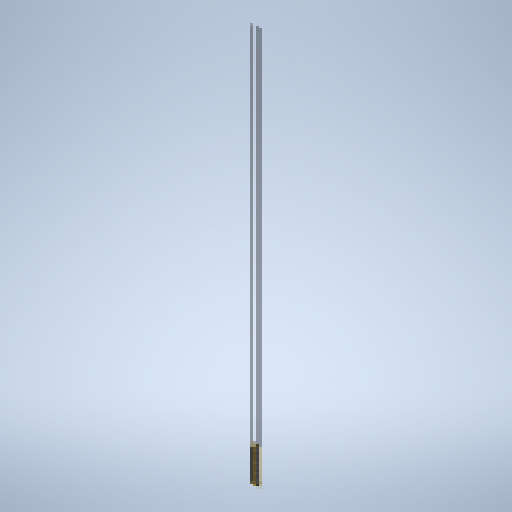
# Autodesk Inventor part: PP0735H(1)
Saved by Autodesk Inventor 2025.2 (Build 292293000, 293)
## iProperties
Category: PARTsolutions
Company: ELDON
Created: 2025-05-02
Part Number: PP0735H(1)
Material: Generic
Catalog Web Link: www.cadenas.de
Description: PP-DIN rails
Vendor: ELDON
Document SubType Name: Modeling
Designer: psAdmin
Manufacturer: ELDON
Mass: 630 g
Surface Area: 1764.71 cm^2
Volume: 84.5125 cm^3
Density: 1 g/cm^3
Appearance: PSOLRGB-175-175-175
PSOL_IDENT_0: {$CADENAS_DATA/23d-libs/eldon/common_pool/accessories/p/pp.prj},167 {VTYP=3D},{NB=PP0735H(1)},{LINA=
PSOL_IDENT_1: PP0735H},{NN=PP},{DATE=04.03.2025 09:38:01},{GEOMDATE=28.02.2025 11:58:07},{VERSION=},{LINEID=1810},
PSOL_IDENT_2: {WBVAR=DETAIL},{WBNUMERIC=DETAIL}  {NB=PP0735H(1)},{LINA=PP0735H},{KT=DUMMY},{ITEM=PP0735H},{DETAIL=
PSOL_IDENT_3: 1},{INFO=Info URL},{DES=Din rail with holes, 2000},{DES1=With holes},{MAT=Galvanized steel},{TYP=Ome
PSOL_IDENT_4: ga},{DIM=7.5 X 35},{HP=Hole pattern 18 x 5.2 mm},{MASS=0.63},{EAN=8713574013193},{TARIFFN=-},{MI=URL
PSOL_IDENT_5: },{MIALG=https://www.eldon.com/catalog-document/PP0515H/mountinginstructions/en/},{INFOPATH=https://
PSOL_IDENT_6: www.nvent.com/en-gb/catalog-document/itemsheet?pid=PP0735H},{V=1},{A=35},{A1=7.5},{A2=4.00},{A3=0.8}
PSOL_IDENT_7: ,{A4=1.8},{A5=0.00},{A6=0.0}
NB: PP0735H(1)
NN: PP
NT: DIN rails
NBSYN: $ITEM.($DETAIL.)
LINA: PP0735H
CATALOG: nVent HOFFMAN IEC-Rated Products
ITEM: PP0735H
DETAIL: high
INFO: Info URL
DES: Din rail with holes, 2000
DES1: With holes
MAT: Galvanized steel
TYP: Omega
DIM: 7.5 X 35
HP: Hole pattern 18 x 5.2 mm
MASS: 0.63
EAN: 8713574013193
MI: URL
SUPPLIER: ELDON
ARTICLENO: PP0735H(1)
BOMINFO: PP0735H
CREATOR: CADENAS GmbH
Title: PP0735H
Author: Cadenas PARTsolutions
Comments: DIN rails
Autodesk Inventor part; units mm, degrees
sketch "Sketch_2" plane through (0, 0, 0) normal (0, 1, 0) x (-1, 0, 0)
  line L0 (14.6744, 3.8205) -> (14.6744, 4.3333)
  line L1 (14.6744, 4.3333) -> (13.0333, 4.3333)
  arc A0 (13.0333, 4.3333) -> (12.1103, 3.4103) centre (13.0333, 3.4103) ccw
  line L2 (12.1103, 3.4103) -> (12.1103, 1.4103)
  arc A1 (11.7, 1) -> (12.1103, 1.4103) centre (11.7, 1.4103) ccw
  line L3 (11.7, 1) -> (-0.3, 1)
  arc A2 (-0.7103, 1.4103) -> (-0.3, 1) centre (-0.3, 1.4103) ccw
  line L4 (-0.7103, 1.4103) -> (-0.7103, 3.4103)
  arc A3 (-0.7103, 3.4103) -> (-1.6333, 4.3333) centre (-1.6333, 3.4103) ccw
  line L5 (-1.6333, 4.3333) -> (-3.2744, 4.3333)
  line L6 (-3.2744, 4.3333) -> (-3.2744, 3.8205)
  line L7 (-3.2744, 3.8205) -> (-1.6333, 3.8205)
  arc A4 (-1.2231, 3.4103) -> (-1.6333, 3.8205) centre (-1.6333, 3.4103) ccw
  line L8 (-1.2231, 3.4103) -> (-1.2231, 1.4103)
  arc A5 (-1.2231, 1.4103) -> (-0.3, 0.4872) centre (-0.3, 1.4103) ccw
  line L9 (-0.3, 0.4872) -> (11.7, 0.4872)
  arc A6 (11.7, 0.4872) -> (12.6231, 1.4103) centre (11.7, 1.4103) ccw
  line L10 (12.6231, 1.4103) -> (12.6231, 3.4103)
  arc A7 (13.0333, 3.8205) -> (12.6231, 3.4103) centre (13.0333, 3.4103) ccw
  line L11 (13.0333, 3.8205) -> (14.6744, 3.8205)
  dimension "d13" = 12
  constraints: 24 end point, 16 point on circle, 8 centre point, 1 parallel
  measures "d13" distance of L3.start L3.end
extrude "Extrusion1" add sketch "Sketch_2" along normal blind 161
sketch "Sketch_6" plane through (0, 0, 0) normal (0, 0, 1) x (1, 0, 0)
  arc A0 (-8.7098, 4.8974) -> (-3.5098, 4.8974) centre (-6.1098, 4.8974) ccw
  line L0 (-3.5098, 4.8974) -> (-3.5098, 17.6974)
  arc A1 (-3.5098, 17.6974) -> (-8.7098, 17.6974) centre (-6.1098, 17.6974) ccw
  line L1 (-8.7098, 17.6974) -> (-8.7098, 4.8974)
  constraints: 4 end point, 4 point on circle, 2 centre point
extrude "Extrusion2" cut sketch "Sketch_6" along normal blind 1
pattern_linear "Rectangular Pattern1" count 80 spacing 23 along (0, 1, 0) of "Extrusion2"
body "Solid1"
